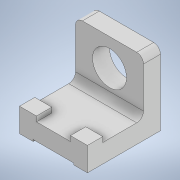
# Autodesk Inventor part: TubeMount
Saved by Autodesk Inventor 2022.2 (Build 262287030, 287C)
## iProperties
Created: 2023-03-13
Part Number: TubeMount
Material: Generic
Document SubType Name: Modeling
Designer: jak27277
Density: 1 g/cm^3
Appearance: Default
Author: jak27277
Autodesk Inventor part; units mm, degrees
ref_plane "YZ Plane" through (0, 0, 0) normal (1, 0, 0) x (0, 1, 0)
ref_plane "XZ Plane" through (0, 0, 0) normal (0, 1, 0) x (-1, 0, 0)
ref_plane "XY Plane" through (0, 0, 0) normal (0, 0, 1) x (1, 0, 0)
sketch "Sketch4" plane through (0, 0, 0) normal (0, 0, 1) x (1, 0, 0)
  circle A0 centre (0, 0) radius 31.75
  line L0 (-63.5, -50.8) -> (63.5, -50.8) construction
  line L1 (63.5, -50.8) -> (63.5, 50.8)
  line L2 (63.5, 50.8) -> (-63.5, 50.8)
  line L3 (-63.5, 50.8) -> (-63.5, -50.8)
  line L4 (-63.5, -50.8) -> (63.5, 50.8) construction
  line L5 (63.5, -50.8) -> (-63.5, 50.8) construction
  line L6 (-63.5, -50.8) -> (63.5, -50.8) construction
  line L7 (63.5, -50.8) -> (63.5, -85.725)
  line L8 (63.5, -85.725) -> (-63.5, -85.725)
  line L9 (-63.5, -85.725) -> (-63.5, -50.8)
  dimension "d2" = 127
  dimension "d3" = 101.6
  dimension "d4" = 63.5
  dimension "d5" = 136.525
  constraints: 20 end point, 4 parallel, 2 horizontal, 2 midpoint, 2 perpendicular, 1 centre point, 1 coincident, 1 collinear
  measures "d2" distance of L1.end L2.end
  measures "d3" distance of L0.end L1.end
  measures "d4" diameter of A0
  measures "d5" distance between parallel lines of L2 L8
extrude "Extrusion1" add sketch "Sketch4" along normal blind 31.75
sketch "Sketch5" plane through (0, 0, 31.75) normal (0, 0, 1) x (1, 0, 0)
  line L0 (-63.5, 50.8) -> (-63.5, -85.725) projected
  line L1 (-63.5, -85.725) -> (63.5, -85.725)
  line L2 (63.5, -85.725) -> (63.5, -41.275)
  line L3 (63.5, -41.275) -> (-63.5, -41.275)
  line L4 (-63.5, -41.275) -> (-63.5, -85.725)
  line L5 (63.5, -85.725) -> (63.5, 50.8) projected
  line L6 (-63.5, -41.275) -> (63.5, -41.275)
  line L7 (63.5, -41.275) -> (63.5, -50.8)
  line L8 (63.5, -50.8) -> (-63.5, -50.8)
  line L9 (-63.5, -50.8) -> (-63.5, -41.275)
  point P0 (0, 0)
  point P1 (-63.5, -50.8)
  dimension "d8" = 44.45
  dimension "d9" = 9.525
  constraints: 16 end point, 4 parallel, 2 horizontal, 2 perpendicular, 1 collinear, 1 point on line
  measures "d8" distance between parallel lines of L1 L3
  measures "d9" distance between parallel lines of L3 L8
extrude "Extrusion2" add sketch "Sketch5" along normal blind 104.775 contours L8 L2 L1 L0
sketch "Sketch6" plane through (0, 0, 136.525) normal (0, 0, 1) x (1, 0, 0)
  line L0 (-63.5, -85.725) -> (63.5, -85.725) projected
  line L1 (-38.1, -85.725) -> (38.1, -85.725)
  line L2 (38.1, -85.725) -> (38.1, -82.55)
  line L3 (38.1, -82.55) -> (-38.1, -82.55)
  line L4 (-38.1, -82.55) -> (-38.1, -85.725)
  line L5 (-63.5, -50.8) -> (-63.5, -85.725) projected
  point P0 (0, 0)
  dimension "d12" = 3.175
  dimension "d13" = 25.4
  dimension "d14" = 76.2
  constraints: 8 end point, 2 parallel, 1 horizontal, 1 perpendicular, 1 point on line
  measures "d12" distance of L3.end L1.start
  measures "d13" distance between parallel lines of L5 L4
  measures "d14" distance of L2.end L3.end
extrude "Extrusion3" cut sketch "Sketch6" against normal through all
sketch "Sketch7" plane through (-63.5, -50.8, 31.75) normal (0, 1, 0) x (1, 0, 0)
  line L0 (127, -104.775) -> (0, -104.775) projected
  line L1 (0, -104.775) -> (31.75, -104.775)
  line L2 (31.75, -104.775) -> (31.75, -76.2)
  line L3 (31.75, -76.2) -> (0, -76.2)
  line L4 (0, -76.2) -> (0, -104.775)
  line L5 (127, 31.75) -> (127, -104.775) projected
  line L6 (95.25, -104.775) -> (127, -104.775)
  line L7 (127, -104.775) -> (127, -76.2)
  line L8 (127, -76.2) -> (95.25, -76.2)
  line L9 (95.25, -76.2) -> (95.25, -104.775)
  line L10 (0, 0) -> (127, 0) projected
  point P0 (63.5, 31.75)
  dimension "d17" = 63.5
  dimension "d18" = 76.2
  constraints: 16 end point, 4 parallel, 2 equal length, 2 horizontal, 2 perpendicular, 2 point on line
  measures "d17" distance between parallel lines of L9 L2
  measures "d18" distance between parallel lines of L10 L8
extrude "Extrusion4" add sketch "Sketch7" along normal blind 9.525
fillet "Fillet1" radius 12.7 3 edges at (63.5, 50.8, 15.875) (-63.5, 50.8, 15.875) (0, -50.8, 31.75)
body "Solid1"
